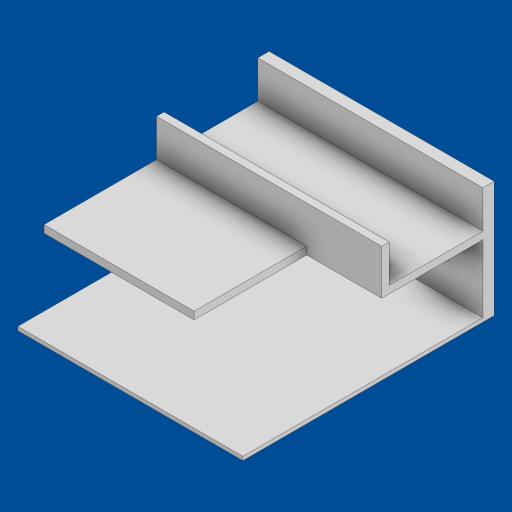
# Autodesk Inventor part: electric_base
Saved by Autodesk Inventor 2023.1 (Build 271208000, 208)
## iProperties
Created: 2023-06-05
Part Number: electric_base
Material: Generic
Document SubType Name: Modeling
Designer: nara atthama
Density: 1 g/cm^3
Appearance: Default
Author: nara atthama
Autodesk Inventor part; units mm, degrees
ref_plane "YZ Plane" through (0, 0, 0) normal (1, 0, 0) x (0, 1, 0)
ref_plane "XZ Plane" through (0, 0, 0) normal (0, 1, 0) x (-1, 0, 0)
ref_plane "XY Plane" through (0, 0, 0) normal (0, 0, 1) x (1, 0, 0)
sketch "Sketch1" plane through (0, 0, 0) normal (0, 1, 0) x (-1, 0, 0)
  line L0 (32.4676, 20.8715) -> (-27.5324, 20.8715)
  line L1 (-27.5324, 20.8715) -> (-27.5324, -46.1285)
  line L2 (-27.5324, -46.1285) -> (32.4676, -46.1285)
  line L3 (32.4676, -46.1285) -> (32.4676, 20.8715)
  point P0 (0, 0)
  dimension "d2" = 60
  dimension "d3" = 67
  constraints: 8 end point, 2 parallel, 1 horizontal, 1 perpendicular
  measures "d2" distance of L0.start L0.end
  measures "d3" distance of L0.end L1.end
extrude "Extrusion1" add sketch "Sketch1" along normal blind 1
sketch "Sketch2" plane through (0, 1, 0) normal (0, 1, 0) x (1, 0, 0)
  line L0 (27.5324, 46.1285) -> (-32.4676, 46.1285) projected
  line L1 (-32.4676, 46.1285) -> (-32.4676, -20.8715) projected
  line L2 (27.5324, 46.1285) -> (-32.4676, 46.1285)
  line L3 (-32.4676, 46.1285) -> (-32.4676, 43.1285)
  line L4 (-32.4676, 43.1285) -> (27.5324, 43.1285)
  line L5 (27.5324, 43.1285) -> (27.5324, 46.1285)
  line L6 (27.5324, 46.1285) -> (24.5324, 46.1285)
  line L7 (24.5324, 46.1285) -> (24.5324, -13.8715)
  line L8 (24.5324, -13.8715) -> (27.5324, -13.8715)
  line L9 (27.5324, -13.8715) -> (27.5324, 46.1285)
  point P0 (0, 0)
  point P1 (24.5324, 43.1285)
  dimension "d8" = 3
  dimension "d9" = 3
  constraints: 16 end point, 4 parallel, 2 horizontal, 2 perpendicular, 1 point on line
  measures "d8" distance between parallel lines of L4 L0
  measures "d9" distance between parallel lines of L9 L7
extrude "Extrusion2" add sketch "Sketch2" along normal blind 20 contours L5 L4 L7 L0 | L7 L4 L1 L0
sketch "Sketch3" plane through (0, 21, 0) normal (0, 1, 0) x (1, 0, 0)
  line L0 (27.5324, 46.1285) -> (-32.4676, 46.1285) projected
  line L1 (-32.4676, 46.1285) -> (-32.4676, 43.1285) projected
  line L2 (-32.4676, 43.1285) -> (27.5324, 43.1285) projected
  line L3 (27.5324, 43.1285) -> (-32.4676, 43.1285) projected
  line L4 (-32.4676, 43.1285) -> (-32.4676, -20.8715) projected
  line L5 (-32.4676, -20.8715) -> (27.5324, -20.8715) projected
  line L6 (27.5324, 46.1285) -> (-32.4676, 46.1285) projected
  line L7 (27.5324, -20.8715) -> (27.5324, 46.1285) projected
  line L8 (-32.4676, 46.1285) -> (27.5324, 46.1285)
  line L9 (27.5324, 46.1285) -> (27.5324, 18.1285)
  line L10 (27.5324, 18.1285) -> (-32.4676, 18.1285)
  line L11 (-32.4676, 18.1285) -> (-32.4676, 46.1285)
  line L12 (-32.4676, 18.1285) -> (27.5324, 18.1285)
  line L13 (27.5324, 18.1285) -> (27.5324, 16.1285)
  line L14 (27.5324, 16.1285) -> (-32.4676, 16.1285)
  line L15 (-32.4676, 16.1285) -> (-32.4676, 18.1285)
  line L16 (27.5324, -20.8715) -> (27.5324, 43.1285) projected
  line L17 (27.5324, 43.1285) -> (27.5324, 46.1285) projected
  line L18 (-32.4676, 16.1285) -> (7.5324, 16.1285)
  line L19 (7.5324, 16.1285) -> (7.5324, -13.8715)
  line L20 (7.5324, -13.8715) -> (-32.4676, -13.8715)
  line L21 (-32.4676, -13.8715) -> (-32.4676, 16.1285)
  point P0 (0, 0)
  point P1 (-32.4676, 16.1285)
  point P2 (-32.4676, 18.1285)
  point P3 (-32.4676, -13.8715)
  dimension "d16" = 2
  dimension "d19" = 25
  dimension "d26" = 40
  dimension "d27" = 30
  constraints: 24 end point, 6 parallel, 3 horizontal, 3 perpendicular, 2 point on line
  measures "d16" distance between parallel lines of L12 L14
  measures "d19" distance between parallel lines of L2 L10
  measures "d26" distance of L19.end L20.end
  measures "d27" distance between parallel lines of L14 L20
extrude "Extrusion3" add sketch "Sketch3" against normal blind 2 contours L7 L10 L4 L2 | L7 L14 L4 L10 | L14 L19 L20 L4
extrude "Extrusion5" add sketch "Sketch3" along normal blind 10 contours L7 L2 L1 L0 | L7 L14 L4 L10
sketch "Sketch5" plane through (27.5324, 0, -46.1285) normal (0, 0, -1) x (-1, 0, 0)
  circle A0 centre (10, 9.9562) radius 1
  circle A1 centre (50, 9.9562) radius 1
  line L0 (0, 0) -> (0, 31) projected
  point P0 (27.5324, 0)
  dimension "d20" = 2
  dimension "d21" = 2
  dimension "d22" = 40
  dimension "d23" = 10
  constraints: 2 centre point, 1 horizontal alignment
  measures "d20" diameter of A0
  measures "d21" diameter of A1
  measures "d22" distance of A1.centre A0.centre
  measures "d23" distance from line of L0 A0.centre
extrude "Extrusion6" cut sketch "Sketch5" against normal blind 20
equation "\"d9\" = d8"
equation "\"d21\" = d20"
body "Solid1"
